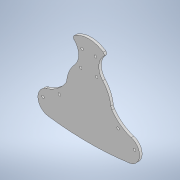
# Autodesk Inventor part: 中間ユニット外
Saved by Autodesk Inventor 2022.2 (Build 262287030, 287C)
## iProperties
Created: 2022-01-03
Part Number: 中間ユニット外
Material: Generic
Document SubType Name: Modeling
Designer: acps
Density: 1 g/cm^3
Appearance: Default
Author: acps
Autodesk Inventor part; units mm, degrees
ref_plane "YZ Plane" through (0, 0, 0) normal (1, 0, 0) x (0, 1, 0)
ref_plane "XZ Plane" through (0, 0, 0) normal (0, 1, 0) x (-1, 0, 0)
ref_plane "XY Plane" through (0, 0, 0) normal (0, 0, 1) x (1, 0, 0)
sketch "Sketch2" plane through (0, 0, 0) normal (0, 0, 1) x (1, 0, 0)
  line L0 (-31.4755, -75) -> (165.3406, -75) construction
  circle A0 centre (7.8339, 40) radius 1.5
  circle A1 centre (7.8339, 40) radius 4.5
  circle A2 centre (7.8339, 40) radius 5.5 construction
  circle A3 centre (35, 0) radius 9 construction
  arc A4 (26.7096, 3.5028) -> (28.866, 26.2368) centre (-8.2942, 18.2924) ccw construction
  arc A5 (44, 47.83) -> (28.866, 26.2368) centre (46.4683, 30) ccw construction
  arc A6 (31.2271, -8.171) -> (58.8706, -11.0424) centre (49.2531, 30.8683) ccw construction
  arc A7 (75.52, -28.3291) -> (58.8706, -11.0424) centre (62.0019, -24.6877) ccw construction
  arc A8 (18.8792, 45.922) -> (16.5694, 19.6548) centre (29.9318, 31.7149) ccw construction
  arc A9 (26.0689, -1.1117) -> (16.5694, 19.6548) centre (-11.6401, -5.8055) ccw construction
  arc A10 (27.6471, -5.1899) -> (50.1513, -21.4983) centre (62.7777, 19.6061) ccw construction
  arc A11 (55.9268, -44.7937) -> (50.1513, -21.4983) centre (46.0404, -34.8812) ccw construction
  arc A12 (17.3547, 44.7312) -> (16.4952, 19.5878) centre (29.9318, 31.7149) ccw
  arc A13 (26.0107, -1.466) -> (16.4952, 19.5878) centre (-11.6401, -5.8055) ccw
  arc A14 (27.3182, -4.8935) -> (50.122, -21.5939) centre (62.7777, 19.6061) ccw
  arc A15 (47.9746, -48.6459) -> (50.122, -21.5939) centre (46.0404, -34.8812) ccw
  circle A16 centre (9.4447, 20) radius 5.5 construction
  circle A17 centre (9.4447, 20) radius 4.5
  circle A18 centre (9.4447, 20) radius 1.5
  circle A19 centre (34.6118, -20) radius 5.5 construction
  circle A20 centre (34.6118, -20) radius 4.5
  circle A21 centre (34.6118, -20) radius 1.5
  circle A22 centre (46.4683, 30) radius 14 construction
  circle A23 centre (29.9318, 31.7149) radius 14 construction
  arc A24 (35.8181, -8.9627) -> (61.1937, 2.3723) centre (31.9094, 33.8592) ccw construction
  arc A25 (84.2559, -4.2737) -> (61.1937, 2.3723) centre (70.7282, -7.8793) ccw construction
  circle A26 centre (53.9309, -32) radius 5.5 construction
  circle A27 centre (53.9309, -32) radius 4.5
  circle A28 centre (53.9309, -32) radius 1.5
  arc A29 (55.4978, -80.8637) -> (53.4691, -79.703) centre (53.6775, -81.6921) ccw
  line L1 (7.8339, 40) -> (7.8339, 30) construction
  arc A30 (17.3547, 44.7312) -> (17, 49) centre (15.4324, 46.7206) ccw
  arc A31 (26.0107, -1.466) -> (27.3182, -4.8935) centre (35, 0) ccw
  line L2 (0, 49) -> (17, 49) construction
  line L3 (-5.664, 54.2816) -> (14.4874, 54.2816) construction
  line L4 (-5.8556, -52) -> (8.6304, -52) construction
  line L5 (0, 49) -> (-17, 49) construction
  line L6 (0, 64.5738) -> (0, -81.6921) construction
  arc A32 (17, 49) -> (-17, 49) centre (0, 24.2816) ccw
  arc A33 (-16.4952, 19.5878) -> (-17.3547, 44.7312) centre (-29.9318, 31.7149) ccw
  circle A34 centre (-7.8339, 40) radius 4.5
  circle A35 centre (-7.8339, 40) radius 1.5
  circle A36 centre (-9.4447, 20) radius 4.5
  circle A37 centre (-9.4447, 20) radius 1.5
  arc A38 (-16.4952, 19.5878) -> (-26.0107, -1.466) centre (11.6401, -5.8055) ccw
  arc A39 (-50.122, -21.5939) -> (-27.3182, -4.8935) centre (-62.7777, 19.6061) ccw
  arc A40 (-27.3182, -4.8935) -> (-26.0107, -1.466) centre (-35, 0) ccw
  circle A41 centre (-34.6118, -20) radius 4.5
  circle A42 centre (-34.6118, -20) radius 1.5
  circle A43 centre (-53.9309, -32) radius 4.5
  circle A44 centre (-53.9309, -32) radius 1.5
  arc A45 (-50.122, -21.5939) -> (-47.9746, -48.6459) centre (-46.0404, -34.8812) ccw
  arc A46 (-17, 49) -> (-17.3547, 44.7312) centre (-15.4324, 46.7206) ccw
  arc A47 (-47.9746, -48.6459) -> (47.9746, -48.6459) centre (0, 292.7765) ccw
  point P0 (28.425, 18.534)
  point P1 (0, 0)
  dimension "d70" = 3
  dimension "d71" = 9
  dimension "d72" = 11
  dimension "d73" = 0.1
  dimension "d74" = 0.1
  dimension "d75" = 75
  dimension "d76" = 3
  dimension "d77" = 9
  dimension "d78" = 11
  dimension "d79" = 20
  dimension "d80" = 40
  dimension "d81" = 3
  dimension "d82" = 9
  dimension "d83" = 11
  dimension "d84" = 20
  dimension "d85" = 3
  dimension "d86" = 9
  dimension "d87" = 11
  dimension "d88" = 32
  dimension "d89" = 2
  dimension "d90" = 10
  dimension "d91" = 0.1
  dimension "d92" = 17
  dimension "d93" = 49
  dimension "d94" = 52
  dimension "d95" = 17
  dimension "d96" = 30
  constraints: 50 point on circle, 48 centre point, 19 symmetric about line, 14 end point, 12 coincident, 10 tangent, 6 horizontal, 3 vertical, 1 concentric, 1 point on line, 29 other
  measures "d70" diameter of A0
  measures "d71" diameter of A1
  measures "d72" diameter of A2
  measures "d73" radial gap between concentric circles of A8 A12
  measures "d74" radial gap between concentric circles of A10 A14
  measures "d75" distance from line of L0 point (0, 0)
  measures "d76" diameter of A18
  measures "d77" diameter of A17
  measures "d78" diameter of A16
  measures "d79" vertical distance of point (0, 0) A16.centre
  measures "d80" vertical distance of point (0, 0) A0.centre
  measures "d81" diameter of A21
  measures "d82" diameter of A20
  measures "d83" diameter of A19
  measures "d84" vertical distance of point (0, 0) A20.centre
  measures "d85" diameter of A28
  measures "d86" diameter of A27
  measures "d87" diameter of A26
  measures "d88" vertical distance of point (0, 0) A26.centre
  measures "d89" radius of A29
  measures "d90" distance of L1.start L1.end
  measures "d91" radial gap between concentric circles of A13 A9
  measures "d92" distance of L5.start L2.end
  measures "d93" distance from line of point (0, 0) L2
  measures "d94" distance from line of point (0, 0) L4
  measures "d95" distance of L5.start L5.end
  measures "d96" radius of A32
extrude "Extrusion2" add sketch "Sketch2" against normal blind 3 contours A1 | A12 A13 A31 A14 A15 A47 A45 A39 A40 A38 A33 A46 A32 A30 | A17 | A20 | A27 | A34 | A36 | A41 | A43
body "Solid2"
